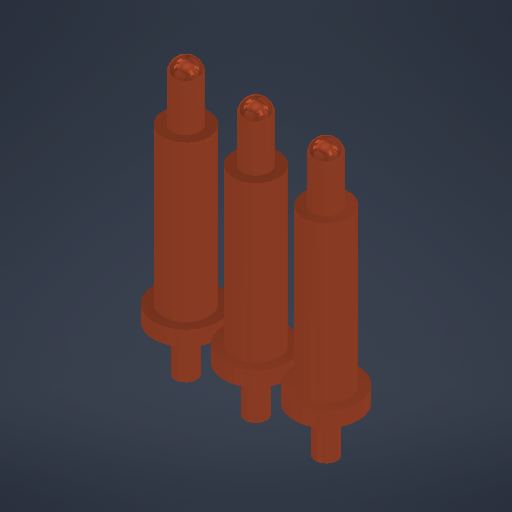
# Autodesk Inventor part: Pogo2
Saved by Autodesk Inventor 2026 (Build 300175000, 175)
## iProperties
Created: 2025-04-17
Part Number: Pogo2
Material: Copper
Document SubType Name: Modeling
Designer: ct_vi
Density: 8.94 g/cm^3
Appearance: Copper - Satin
Author: ct_vi
Autodesk Inventor part; units mm, degrees
ref_plane "YZ Plane" through (0, 0, 0) normal (1, 0, 0) x (0, 1, 0)
ref_plane "XZ Plane" through (0, 0, 0) normal (0, 1, 0) x (-1, 0, 0)
sketch "Sketch1" plane through (0, 0, 0) normal (0, 1, 0) x (-1, 0, 0)
  line L0 (-8.55, 0) -> (-8.55, 0)
  line L1 (5.4, 2.35) -> (-5.4, 2.35)
  line L2 (-7.75, 0) -> (-7.75, 0)
  line L3 (7.75, 0) -> (7.75, 0)
  arc A0 (-5.4, 2.35) -> (-7.75, 0) centre (-5.4, 0) ccw
  arc A1 (-7.75, 0) -> (-5.4, -2.35) centre (-5.4, 0) ccw
  arc A2 (7.75, 0) -> (5.4, 2.35) centre (5.4, 0) ccw
  arc A3 (5.4, -2.35) -> (7.75, 0) centre (5.4, 0) ccw
  circle A4 centre (5.4, 0) radius 1.5
  circle A5 centre (-5.4, 0) radius 1.5
  circle A6 centre (2.3, 0) radius 0.75
  circle A7 centre (0, 0) radius 0.75
  circle A8 centre (-2.3, 0) radius 0.75
  circle A9 centre (2.3, 0) radius 0.35
  circle A10 centre (0, 0) radius 0.35
  circle A11 centre (-2.3, 0) radius 0.45
  line L4 (-15.2366, 19.4813) -> (26.8433, 19.4813) construction
  line L5 (26.8433, 19.4813) -> (26.8433, -5.0467) construction
  line L6 (26.8433, -5.0467) -> (-15.2366, -5.0467) construction
  line L7 (-15.2366, -5.0467) -> (-15.2366, 19.4813) construction
  line L8 (-8.3717, -2.35) -> (8.3717, -2.35)
  line L9 (8.3717, 2.35) -> (-8.3717, 2.35)
  circle A12 centre (2.3, 0) radius 1.05
  circle A13 centre (0, 0) radius 1.05
  circle A14 centre (-2.3, 0) radius 1.05
  circle A15 centre (-2.3, 0) radius 0.35
  circle A16 centre (0, 0) radius 0.45
  circle A17 centre (2.3, 0) radius 0.45
  point P0 (7.75, 0)
  point P1 (-5.4, -2.35)
  point P2 (5.4, -2.35)
  dimension "d5" = 2.35
  dimension "d6" = 3
  dimension "d7" = 3
  dimension "d10" = 1.5
  dimension "d11" = 4.6
  dimension "d14" = 0.9
  dimension "d201" = 2.1
  dimension "d202" = 2.1
  dimension "d203" = 2.1
  dimension "d204" = 1.5
  dimension "d205" = 1.5
  dimension "d213" = 0.7
  dimension "d214" = 0.9
  dimension "d215" = 0.9
  constraints: 18 centre point, 12 end point, 8 coincident, 8 point on circle, 6 tangent, 3 equal radius, 2 horizontal, 2 parallel, 1 perpendicular, 2 other
  measures "d5" radius of A0
  measures "d6" diameter of A4
  measures "d7" diameter of A5
  measures "d10" diameter of A8
  measures "d11" distance of A8.centre A6.centre
  measures "d14" diameter of A11
  measures "d201" diameter of A12
  measures "d202" diameter of A13
  measures "d203" diameter of A14
  measures "d204" diameter of A7
  measures "d205" diameter of A6
  measures "d213" diameter of A15
  measures "d214" diameter of A16
  measures "d215" diameter of A17
ref_plane "Work Plane2" through (-5.4, 0, 2.35) normal (0, 0, 1) x (1, 0, 0)
sketch "Sketch3" plane through (-5.4, 0, 2.35) normal (0, 0, 1) x (1, 0, 0)
  line L0 (-9.7661, 9.6728) -> (32.2033, 9.6728) construction
  line L1 (32.2033, 9.6728) -> (32.2033, -14.7908) construction
  line L2 (32.2033, -14.7908) -> (-9.7661, -14.7908) construction
  line L3 (-9.7661, -14.7908) -> (-9.7661, 9.6728) construction
  point P0 (5.4, 0)
  constraints: 2 other
extrude "Extrusion9" add sketch "Sketch1" along normal blind 0.5 contours A6 | A7 | A8 | A9 | A10 | A11 | A12 | A13 | A14 | A15 | A16 | A17
extrude "Extrusion10" add sketch "Sketch1" against normal blind 1.5 contours A9 | A10 | A15
extrude "Extrusion11" add sketch "Sketch1" along normal blind 5.6 contours A6 | A7 | A8 | A9 | A10 | A11 | A15 | A16 | A17
extrude "Extrusion12" add sketch "Sketch1" along normal blind 7.5 contours A9 | A10 | A11 | A15 | A16 | A17
fillet "Fillet1" radius 0.45 3 edges at (2.75, 7.5, 0) (0.45, 7.5, 0) (-1.85, 7.5, 0)
body "Solid2"
